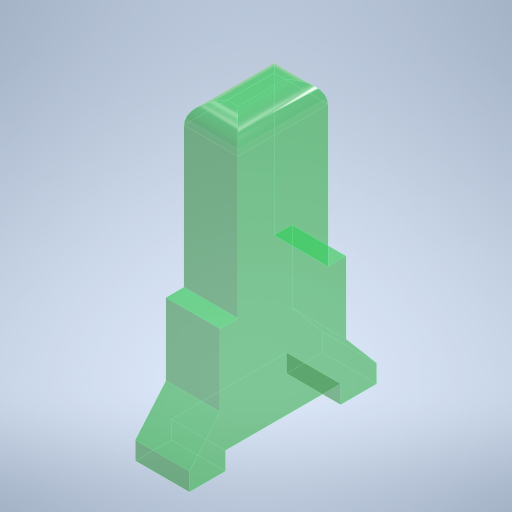
# Autodesk Inventor part: LightPipe
Saved by Autodesk Inventor 2024 (Build 280153000, 153)
## iProperties
Created: 2024-03-14
Part Number: LightPipe
Material: Generic
Document SubType Name: Modeling
Designer: Jonat
Density: 1 g/cm^3
Appearance: Clear - Green 1
Author: Jonat
Autodesk Inventor part; units mm, degrees
ref_plane "YZ Plane" through (0, 0, 0) normal (1, 0, 0) x (0, 1, 0)
ref_plane "XZ Plane" through (0, 0, 0) normal (0, 1, 0) x (-1, 0, 0)
ref_plane "XY Plane" through (0, 0, 0) normal (0, 0, 1) x (1, 0, 0)
sketch "Sketch1" plane through (0, 0, 0) normal (0, 1, 0) x (-1, 0, 0)
  line L0 (-0.75, -1.6) -> (0.75, -1.6)
  line L1 (0.75, -1.6) -> (0.75, 1.6)
  line L2 (0.75, 1.6) -> (-0.75, 1.6)
  line L3 (-0.75, 1.6) -> (-0.75, -1.6)
  line L4 (-0.75, -1.6) -> (0.75, 1.6) construction
  line L5 (0.75, -1.6) -> (-0.75, 1.6) construction
  line L6 (0.75, 1.6) -> (-0.75, 1.6)
  line L7 (-0.75, 1.6) -> (-0.75, 2.6)
  line L8 (-0.75, 2.6) -> (0.75, 2.6)
  line L9 (0.75, 2.6) -> (0.75, 1.6)
  line L10 (-0.75, -1.6) -> (0.75, -1.6)
  line L11 (0.75, -1.6) -> (0.75, -2.6)
  line L12 (0.75, -2.6) -> (-0.75, -2.6)
  line L13 (-0.75, -2.6) -> (-0.75, -1.6)
  point P0 (0, 0)
  point P1 (0.75, -1.6)
  dimension "d0" = 3.2
  dimension "d1" = 1.5
  dimension "d2" = 1
  dimension "d3" = 1
  constraints: 28 end point, 6 parallel, 3 horizontal, 3 perpendicular, 2 midpoint, 1 point on line
  measures "d0" distance between parallel lines of L0 L2
  measures "d1" distance between parallel lines of L3 L1
  measures "d2" distance of L6.end L7.end
  measures "d3" distance of L12.end L0.start
extrude "Extrusion1" add sketch "Sketch1" along normal blind 0.5 contours L0 L11 L12 L13 | L7 L8 L9 L2
sketch "Sketch2" plane through (0.75, 0, 2.6) normal (1, 0, 0) x (0, 0, -1)
  line L0 (0, 0.5) -> (1, 0.5) projected
  line L1 (0.85, 0.5) -> (4.35, 0.5)
  line L2 (4.35, 0.5) -> (4.35, 1.5)
  line L3 (4.35, 1.5) -> (0.85, 1.5)
  line L4 (0.85, 1.5) -> (0.85, 0.5)
  line L5 (0.85, 1.5) -> (0, 0.5)
  line L6 (5.2, 0) -> (5.2, 0.5) projected
  line L7 (4.35, 1.5) -> (5.2, 0.5)
  line L8 (0, 0) -> (1, 0) construction
  line L9 (0, 0) -> (5.2, 0) construction
  line L10 (2.6, 0) -> (2.6, 2.5684) construction
  line L11 (0, 0.5) -> (5.2, 0.5)
  point P0 (2.6, 0.5)
  dimension "d10" = 3.5
  dimension "d19" = 1
  constraints: 18 end point, 2 horizontal, 2 midpoint, 2 parallel, 2 point on line, 1 collinear, 1 perpendicular, 1 vertical
  measures "d10" distance of L3.end L2.end
  measures "d19" distance between parallel lines of L1 L3
extrude "Extrusion3" add sketch "Sketch2" against normal blind 1.5
sketch "Sketch5" plane through (0.75, 1.5, 1.75) normal (0, 1, 0) x (1, 0, 0)
  line L0 (-1.5, 0) -> (-1.5, 3.5) projected
  line L1 (0, 3.5) -> (0, 0) projected
  line L2 (-1.5, 3.5) -> (0, 3.5)
  line L3 (0, 3.5) -> (0, 0)
  line L4 (0, 0) -> (-1.5, 0)
  line L5 (-1.5, 0) -> (-1.5, 3.5)
  point P0 (-0.75, 1.75)
  point P1 (0, 3.5)
  point P2 (-1.5, 0)
  constraints: 8 end point, 2 parallel, 1 horizontal, 1 perpendicular
extrude "Extrusion5" add sketch "Sketch5" along normal blind 2
sketch "Sketch6" plane through (0.75, 3.5, 1.75) normal (0, 1, 0) x (1, 0, 0)
  line L0 (-1.5, 3) -> (0, 3)
  line L1 (0, 3) -> (0, 0.5)
  line L2 (0, 0.5) -> (-1.5, 0.5)
  line L3 (-1.5, 0.5) -> (-1.5, 3)
  line L4 (0, 0) -> (0, 3.5) construction
  line L5 (0, 0) -> (0, 0.5) construction
  line L6 (-0.75, 3) -> (-0.75, 3.5) construction
  line L7 (0, 3.5) -> (-1.5, 3.5) construction
  line L8 (-0.75, 0.5) -> (-0.75, 0) construction
  point P0 (-0.75, 1.75)
  point P1 (-1.5, 1.75)
  point P2 (0, 1.75)
  dimension "d20" = 2.5
  constraints: 14 end point, 5 midpoint, 2 parallel, 2 perpendicular, 1 collinear, 1 horizontal, 1 point on line
  measures "d20" distance of L0.end L1.end
extrude "Extrusion6" add sketch "Sketch6" along normal blind 4.5
fillet "Fillet1" radius 0.6 4 edges at (0, 8, -1.25) (-0.75, 8, 0) (0, 8, 1.25) (0.75, 8, 0)
sketch "Sketch4" plane through (0.75, 1.5, 1.75) normal (0, 1, 0) x (1, 0, 0)
  line L0 (-1.5, 3) -> (0, 3)
  line L1 (0, 3) -> (0, 0.5)
  line L2 (0, 0.5) -> (-1.5, 0.5)
  line L3 (-1.5, 0.5) -> (-1.5, 3)
  line L4 (-1.5, 0) -> (-1.5, 3.5) projected
  line L5 (0, 3.5) -> (0, 0) projected
  line L6 (0, 3.5) -> (-1.5, 3.5) projected
  point P0 (-0.75, 1.75)
  point P1 (-1.5, 1.75)
  point P2 (0, 1.75)
  point P3 (-0.75, 3)
  dimension "d13" = 2.5
  dimension "d14" = 0.5
  constraints: 8 end point, 5 midpoint, 2 parallel, 1 horizontal, 1 perpendicular
  measures "d13" distance of L0.end L1.end
  measures "d14" distance from line of point (-0.75, 3) L6
body "Solid1"
